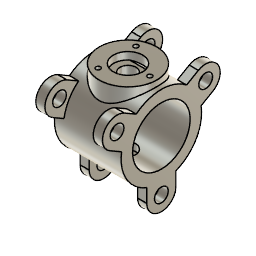
38 (Autodesk Fusion 360 design; units mm, degrees)
Autodesk Fusion 360 part; units mm, degrees
note: some values were not read from the file. Set by a fixed rule: which face or edge a step refers to.
sketch "草图1" plane through (0, 0, 0) normal (1, 0, 0) x (0, 1, 0)
  circle A0 centre (0, 0) radius 25
  circle A1 centre (0, -44.45) radius 6
  line L0 (-12.7, -44.45) -> (-12.7, -32.6146)
  line L1 (12.7, -44.45) -> (12.7, -32.6146)
  line L2 (0, 100) -> (0, -200) construction
  arc A2 (-12.7, -44.45) -> (12.7, -44.45) centre (0, -44.45) ccw
  line L3 (32.1448, 33.2235) -> (21.895, 27.3058)
  line L4 (44.8448, 11.2265) -> (34.595, 5.3088)
  circle A3 centre (38.4948, 22.225) radius 6
  arc A4 (44.8448, 11.2265) -> (32.1448, 33.2235) centre (38.4948, 22.225) ccw
  line L5 (-44.8448, 11.2265) -> (-34.595, 5.3088)
  line L6 (-32.1448, 33.2235) -> (-21.895, 27.3058)
  circle A5 centre (-38.4948, 22.225) radius 6
  arc A6 (-32.1448, 33.2235) -> (-44.8448, 11.2265) centre (-38.4948, 22.225) ccw
  arc A7 (21.895, 27.3058) -> (-21.895, 27.3058) centre (0, 0) ccw
  arc A8 (-34.595, 5.3088) -> (-12.7, -32.6146) centre (0, 0) ccw
  arc A9 (12.7, -32.6146) -> (34.595, 5.3088) centre (0, 0) ccw
  dimension "d1" = 44.45
  dimension "d2" = 70
  dimension "d3" = 50
  dimension "d4" = 12.7
  dimension "d5" = 12
  dimension "d7" = 360
  constraint coincident A0.centre A7.centre
  constraint concentric A1 A2
  constraint coincident L0.end A7
  constraint tangent L0 A2
  constraint coincident L1.end A7
  constraint tangent L1 A2
  constraint vertical L2
  constraint collinear A1.centre L2.start L2.end
  constraint parallel L0 L2
  constraint parallel L1 L2
  constraint concentric A7 A8
  constraint concentric A8 A9
  measures "d1" distance of A0.centre A1.centre
  measures "d2" diameter of A7
  measures "d3" diameter of A0
  measures "d4" radius of A2
  measures "d5" diameter of A1
extrude "拉伸1" add sketch "草图1" along normal blind 8 makes body 1
copy_body "复制和粘贴实体1" bodies 1 makes body 2
move_body "移动1" bodies 2 to x (1, 0, 0) y (0, 1, 0) z (0, 0, 1) at (-50, 0, 0)
sketch "草图2" plane through (0, 0, 0) normal (1, 0, 0) x (0, 1, 0)
  circle A0 centre (0, 0) radius 25
  circle A1 centre (0, 0) radius 35
  dimension "d10" = 70
  dimension "d11" = 50
  constraint coincident A0.centre A1.centre
  measures "d10" diameter of A1
  measures "d11" diameter of A0
extrude "拉伸2" add sketch "草图2" against normal blind 42 separate body makes body 3
ref_plane "工作平面1" through (0, 0, 40) normal (0, 0, 1) x (1, 0, 0)
sketch "草图3" plane through (0, 0, 40) normal (0, 0, 1) x (1, 0, 0)
  circle A0 centre (-21, 0) radius 25
  circle A1 centre (-21, 0) radius 12.7
  circle A2 centre (-21, 0) radius 7
  circle A3 centre (-2, 0) radius 2
  line L0 (-90, 0) -> (40, 0) construction
  circle A4 centre (-30.5, 16.4545) radius 2
  circle A5 centre (-30.5, -16.4545) radius 2
  dimension "d15" = 14
  dimension "d16" = 25.4
  dimension "d17" = 50
  dimension "d18" = 4
  dimension "d19" = 21
  dimension "d20" = 19
  dimension "d22" = 360
  constraint concentric A0 A1
  constraint concentric A1 A2
  constraint horizontal L0
  constraint collinear A3.centre L0.start L0.end
  constraint collinear A0.centre A3.centre L0.end
  measures "d15" diameter of A2
  measures "d16" diameter of A1
  measures "d17" diameter of A0
  measures "d18" diameter of A3
  measures "d19" distance of origin A0.centre
  measures "d20" distance of A0.centre A3.centre
combine "合并1" operation add target body 1 tool bodies 2 3
extrude "拉伸3" add sketch "草图3" along normal up to surface contours A0 end surface at (-28, 28.3162, -20.5717) on bodies 1 bodies 1
extrude "拉伸4" cut sketch "草图3" along normal up to surface contours A3 | A4 | A5 end surface at (-11.3333, -24.9689, -1.2461) on bodies 1 bodies 1
extrude "拉伸5" cut sketch "草图3" against normal blind 6.35 contours A1 bodies 1
extrude "拉伸6" cut sketch "草图3" against normal blind 63.66 contours A2 bodies 1
extrude "拉伸7" cut sketch "草图3" against normal blind 70.01 contours A2 bodies 1
equation "d1 = ( 88.9 / 2 ) * 1 mm"
equation "d31 = -63.66 mm - 6.35 mm"
